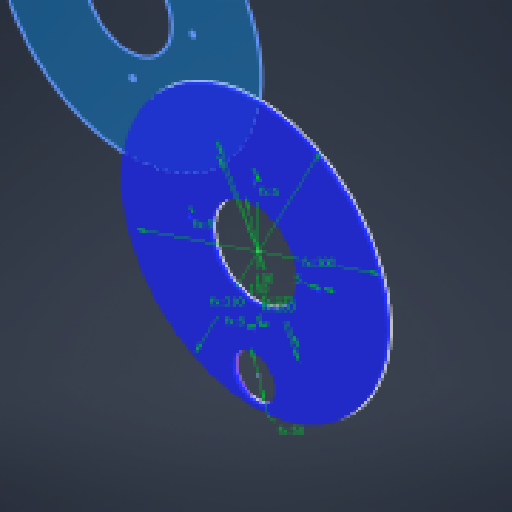
# Autodesk Inventor part: Part1
Saved by Autodesk Inventor 2027.1 (Build 311270010, 270A)
## iProperties
Created: 2026-09-28
Part Number: Part1
Material: Steel, Paint Finish, Blue
Document SubType Name: Modeling
Designer: daniel
Density: 7.85 g/cm^3
Appearance: Blue - Wall Paint - Glossy
Mass: 2574.04 g
Surface Area: 1387.01 cm^2
Volume: 327.904 cm^3
Author: daniel
Autodesk Inventor part; units mm, degrees
ref_plane "YZ Plane" through (0, 0, 0) normal (1, 0, 0) x (0, 1, 0)
ref_plane "XZ Plane" through (0, 0, 0) normal (0, 1, 0) x (-1, 0, 0)
ref_plane "XY Plane" through (0, 0, 0) normal (0, 0, 1) x (1, 0, 0)
sketch "Sketch1" plane through (0, 0, 0) normal (0, 0, 1) x (1, 0, 0)
  circle A0 centre (0, 0) radius 150
  circle A1 centre (0, 0) radius 100
  circle A2 centre (0, 0) radius 155
  circle A3 centre (0, -125) radius 25
  circle A4 centre (0, 0) radius 87.5
  circle A5 centre (0, 0) radius 75
  circle A6 centre (0, 0) radius 50
  circle A7 centre (75, 0) radius 2.5
  circle A8 centre (0, -75) radius 2.5
  circle A9 centre (0, 75) radius 2.5
  circle A10 centre (-75, 0) radius 2.5
  point P0 (0, -150)
  point P1 (0, -100)
  dimension "d0" = 300
  dimension "d1" = 200
  dimension "d2" = 310
  dimension "d3" = 50
  dimension "d8" = 175
  dimension "d9" = 150
  dimension "d10" = 100
  dimension "d11" = 5
  dimension "d12" = 5
  dimension "d13" = 5
  dimension "d14" = 5
  constraints: 11 centre point, 6 coincident, 4 point on circle, 1 tangent
  measures "d0" diameter of A0
  measures "d1" diameter of A1
  measures "d2" diameter of A2
  measures "d3" diameter of A3
  measures "d8" diameter of A4
  measures "d9" diameter of A5
  measures "d10" diameter of A6
  measures "d11" diameter of A7
  measures "d12" diameter of A8
  measures "d13" diameter of A9
  measures "d14" diameter of A10
extrude "Extrusion1" add sketch "Sketch1" along normal blind 5 contours A1 | A0 | A2 | A4 | A7 A5 A8 A10 A9
equation "\"d0\" = 6 * Product_dia"
equation "\"d1\" = 4 * Product_dia"
equation "\"d3\" = Product_dia"
equation "\"d8\" = 3.5 * Product_dia"
equation "\"d12\" = d11"
equation "\"d13\" = d11"
equation "\"d14\" = d11"
equation "\"Product_dia\" = 50"
equation "\"GridTotalSize\" = 63"
equation "\"GridBorderThickness\" = 5"
equation "\"GridBorderFillets\" = 7"
equation "\"BaseTotalWidth\" = 352"
equation "\"GridProcutClearance\" = 3"
equation "\"ProductBaseHeight\" = 35"
body "Solid1"
